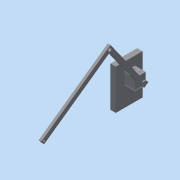
# Autodesk Inventor part: horizontal
Saved by Autodesk Inventor 2019 (Build 230136000, 136)
## iProperties
Created: 2020-02-18
Part Number: horizontal
Material: Generic
Document SubType Name: Modeling
Designer: Sudhanshu
Density: 1 g/cm^3
Appearance: Default
Author: Sudhanshu
Autodesk Inventor part; units mm, degrees
ref_plane "YZ Plane" through (0, 0, 0) normal (1, 0, 0) x (0, 1, 0)
ref_plane "XZ Plane" through (0, 0, 0) normal (0, 1, 0) x (-1, 0, 0)
ref_plane "XY Plane" through (0, 0, 0) normal (0, 0, 1) x (1, 0, 0)
sketch "Sketch1" plane through (0, 0, 0) normal (1, 0, 0) x (0, 1, 0)
  line L0 (0, 0) -> (-150, 0)
  line L1 (-150, 0) -> (-150, -100)
  line L2 (-150, -100) -> (0, -100)
  line L3 (0, -100) -> (0, 0)
  dimension "d0" = 150
  dimension "d1" = 100
  constraints: 8 end point, 2 parallel, 1 horizontal, 1 perpendicular
  measures "d0" distance of L2.end L1.end
  measures "d1" distance of L1.end L0.end
extrude "Extrusion1" add sketch "Sketch1" along normal blind 20
sketch "Sketch2" plane through (20, 0, 0) normal (1, 0, 0) x (0, 0, -1)
  line L0 (32.1942, -72.8605) -> (72.1942, -72.8605)
  line L1 (72.1942, -72.8605) -> (72.1942, -32.8605)
  line L2 (72.1942, -32.8605) -> (32.1942, -32.8605)
  line L3 (32.1942, -32.8605) -> (32.1942, -72.8605)
  point P0 (0, 0)
  dimension "d4" = 40
  dimension "d5" = 40
  constraints: 8 end point, 2 parallel, 1 horizontal, 1 perpendicular
  measures "d4" distance of L2.end L1.end
  measures "d5" distance of L1.end L0.end
extrude "Extrusion2" add sketch "Sketch2" along normal blind 40
sketch "Sketch3" plane through (60, 0, 0) normal (1, 0, 0) x (0, 0, -1)
  line L0 (32.1942, -72.8605) -> (32.1942, -32.8605) projected
  line L1 (32.1942, -72.8605) -> (32.1942, -32.8605)
  line L2 (32.1942, -32.8605) -> (32.1942, -52.8605)
  line L3 (48.2142, -59.6131) -> (57.4566, -59.6131)
  line L4 (57.4566, -59.6131) -> (57.4566, -46.3658)
  line L5 (57.4566, -46.3658) -> (48.2142, -46.3658)
  line L6 (48.2142, -46.3658) -> (48.2142, -59.6131)
  point P0 (0, 0)
  constraints: 12 end point, 2 parallel, 1 horizontal, 1 midpoint, 1 perpendicular, 1 vertical
extrude "Extrusion3" add sketch "Sketch3" along normal blind 15
sketch "Sketch4" plane through (60, 0, 0) normal (1, 0, 0) x (0, 0, -1)
  point P0 (0, 0)
sketch "Sketch5" plane through (60, 0, 0) normal (1, 0, 0) x (0, 0, -1)
  line L0 (57.1037, -71.8566) -> (71.8566, -60.4104)
  line L1 (71.8566, -60.4104) -> (45.9119, -32.8605)
  line L2 (32.1942, -32.8605) -> (72.1942, -32.8605) projected
  line L3 (33.6968, -44.3638) -> (57.1037, -71.8566)
  line L4 (32.1942, -42.5989) -> (45.9119, -32.8605)
  line L5 (32.1942, -42.5989) -> (57.1037, -71.8566)
  point P0 (0, 0)
  constraints: 10 end point, 4 point on line
extrude "Extrusion4" add sketch "Sketch5" along normal blind 10
sketch "Sketch6" plane through (60, -42.5989, -32.1942) normal (0, 0.8154167, 0.5788745) x (1, 0, 0)
  line L0 (0, 16.823) -> (10, 16.823) projected
  line L1 (0, 0) -> (10, 0) projected
  line L2 (10, 16.823) -> (0, 16.823)
  line L3 (0, 16.823) -> (0, 0)
  line L4 (0, 0) -> (10, 0)
  line L5 (10, 0) -> (10, 16.823)
  point P0 (-60, -1.5923)
  constraints: 8 end point, 2 parallel, 1 horizontal, 1 perpendicular
extrude "Extrusion5" add sketch "Sketch6" along normal blind 200
sketch "Sketch7" plane through (60, -42.5989, -32.1942) normal (0, -0.5788745, 0.8154167) x (1, 0, 0)
  line L0 (10, 0) -> (10, 200) projected
  line L1 (0, 0) -> (0, 200) projected
  line L2 (10, 200) -> (0, 200)
  line L3 (0, 200) -> (0, 182.714)
  line L4 (0, 182.714) -> (10, 182.714)
  line L5 (10, 182.714) -> (10, 200)
  point P0 (-60, 53.3722)
  constraints: 8 end point, 2 parallel, 1 horizontal, 1 perpendicular, 1 point on line
extrude "Extrusion6" add sketch "Sketch7" along normal blind 300
sketch "Sketch8" plane through (70, 0, 0) normal (1, 0, 0) x (0, 0, -1)
  point P0 (0, 0)
sketch "Sketch9" plane through (70, 0, 0) normal (1, 0, 0) x (0, 0, -1)
  circle A0 centre (-71.8205, 116.6834) radius 6.7198
  point P0 (0, 0)
  constraints: 1 centre point
extrude "Extrusion7" cut sketch "Sketch9" along normal through all both and the other way through all
sketch "Sketch10" plane through (70, 0, 0) normal (1, 0, 0) x (0, 0, -1)
  point P0 (0, 0)
sketch "Sketch11" plane through (70, 0, 0) normal (1, 0, 0) x (0, 0, -1)
  circle A0 centre (-318.1993, -56.6737) radius 3.8597
  point P0 (0, 0)
  constraints: 1 centre point
extrude "Extrusion8" cut sketch "Sketch11" along normal through all both and the other way through all
sketch "Sketch16" plane through (20, 0, 0) normal (1, 0, 0) x (0, 0, -1)
  point P0 (0, 0)
sketch "Sketch17" plane through (20, 0, 0) normal (1, 0, 0) x (0, 0, -1)
  line L0 (32.6643, -74.5991) -> (72.9814, -74.5991)
  line L1 (72.9814, -74.5991) -> (72.9814, -77.9588)
  line L2 (72.9814, -77.9588) -> (32.6643, -77.9588)
  line L3 (32.6643, -77.9588) -> (32.6643, -74.5991)
  point P0 (0, 0)
  constraints: 8 end point, 2 parallel, 1 horizontal, 1 perpendicular
extrude "Extrusion9" add sketch "Sketch17" along normal blind 40
sketch "Sketch18" plane through (20, -77.9588, -72.9814) normal (0, -1, 0) x (1, 0, 0)
  line L0 (0, 0.7872) -> (40, 0.7872) projected
  line L1 (40, 40.3171) -> (40, 0.7872)
  line L2 (40, 0.7872) -> (0, 0.7872)
  line L3 (0, 0.7872) -> (0, 40.3171)
  line L4 (0, 40.3171) -> (40, 40.3171)
  line L5 (40, 40.3171) -> (40, 0) projected
  line L6 (40, 20.1585) -> (0, 20.5522)
  line L7 (20, 40.3171) -> (20, 0)
  line L8 (0, 0) -> (40, 0) projected
  line L9 (40, 40.3171) -> (20, 40.3171)
  line L10 (30, 40.3171) -> (20, 40.3171)
  line L11 (0, 40.3171) -> (40, 40.3171) projected
  line L12 (0, 40.3171) -> (20, 40.3171)
  circle A0 centre (30, 30.5773) radius 1.5
  circle A1 centre (30, 11.3652) radius 1.5
  circle A2 centre (8.8768, 11.3652) radius 1.5
  circle A3 centre (8.8768, 30.5773) radius 1.5
  point P0 (-20, 72.9814)
  dimension "d22" = 3
  dimension "d23" = 3
  dimension "d24" = 3
  dimension "d25" = 3
  constraints: 18 end point, 5 midpoint, 4 centre point, 3 collinear, 3 perpendicular, 1 vertical
  measures "d22" diameter of A0
  measures "d23" diameter of A1
  measures "d24" diameter of A2
  measures "d25" diameter of A3
extrude "Extrusion10" cut sketch "Sketch18" along normal through all both and the other way through all contours A0 | A1 | A2 | A3
body "Solid1"
